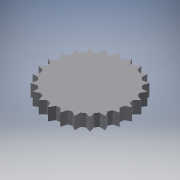
# Autodesk Inventor part: Piñon_1
Saved by Autodesk Inventor 2017 (Build 210142000, 142)
## iProperties
Part Number: Piñon_1
Material: Genérico
Document SubType Name: Modeling
Designer: Daniel Caycedo
Density: 1 g/cm^3
Appearance: Valor por defecto
Author: Daniel Caycedo
Autodesk Inventor part; units mm, degrees
ref_plane "YZ Plane" through (0, 0, 0) normal (1, 0, 0) x (0, 1, 0)
ref_plane "XZ Plane" through (0, 0, 0) normal (0, 1, 0) x (-1, 0, 0)
ref_plane "XY Plane" through (0, 0, 0) normal (0, 0, 1) x (1, 0, 0)
sketch "Boceto1" plane through (0, 0, 0) normal (0, 0, 1) x (1, 0, 0)
  circle A0 centre (0, 0) radius 15
  line L0 (0, 0) -> (0, 15)
  line L1 (0, 15) -> (0, 14)
  line L2 (-1.7321, 14) -> (0, 17)
  line L3 (0, 17) -> (1.7321, 14)
  line L4 (1.7321, 14) -> (-1.7321, 14)
  line L5 (-5.2965, 13.0747) -> (-4.3999, 16.4207)
  line L6 (-1.9504, 13.9712) -> (-5.2965, 13.0747)
  line L7 (-4.3999, 16.4207) -> (-1.9504, 13.9712)
  line L8 (-8.5, 11.2583) -> (-8.5, 14.7224)
  line L9 (-5.5, 12.9904) -> (-8.5, 11.2583)
  line L10 (-8.5, 14.7224) -> (-5.5, 12.9904)
  line L11 (-11.1242, 8.6748) -> (-12.0208, 12.0208)
  line L12 (-8.6748, 11.1242) -> (-11.1242, 8.6748)
  line L13 (-12.0208, 12.0208) -> (-8.6748, 11.1242)
  line L14 (-12.9904, 5.5) -> (-14.7224, 8.5)
  line L15 (-11.2583, 8.5) -> (-12.9904, 5.5)
  line L16 (-14.7224, 8.5) -> (-11.2583, 8.5)
  line L17 (-13.9712, 1.9504) -> (-16.4207, 4.3999)
  line L18 (-13.0747, 5.2965) -> (-13.9712, 1.9504)
  line L19 (-16.4207, 4.3999) -> (-13.0747, 5.2965)
  line L20 (-14, -1.7321) -> (-17, 0)
  line L21 (-14, 1.7321) -> (-14, -1.7321)
  line L22 (-17, 0) -> (-14, 1.7321)
  line L23 (-13.0747, -5.2965) -> (-16.4207, -4.3999)
  line L24 (-13.9712, -1.9504) -> (-13.0747, -5.2965)
  line L25 (-16.4207, -4.3999) -> (-13.9712, -1.9504)
  line L26 (-11.2583, -8.5) -> (-14.7224, -8.5)
  line L27 (-12.9904, -5.5) -> (-11.2583, -8.5)
  line L28 (-14.7224, -8.5) -> (-12.9904, -5.5)
  line L29 (-8.6748, -11.1242) -> (-12.0208, -12.0208)
  line L30 (-11.1242, -8.6748) -> (-8.6748, -11.1242)
  line L31 (-12.0208, -12.0208) -> (-11.1242, -8.6748)
  line L32 (-5.5, -12.9904) -> (-8.5, -14.7224)
  line L33 (-8.5, -11.2583) -> (-5.5, -12.9904)
  line L34 (-8.5, -14.7224) -> (-8.5, -11.2583)
  line L35 (-1.9504, -13.9712) -> (-4.3999, -16.4207)
  line L36 (-5.2965, -13.0747) -> (-1.9504, -13.9712)
  line L37 (-4.3999, -16.4207) -> (-5.2965, -13.0747)
  line L38 (1.7321, -14) -> (0, -17)
  line L39 (-1.7321, -14) -> (1.7321, -14)
  line L40 (0, -17) -> (-1.7321, -14)
  line L41 (5.2965, -13.0747) -> (4.3999, -16.4207)
  line L42 (1.9504, -13.9712) -> (5.2965, -13.0747)
  line L43 (4.3999, -16.4207) -> (1.9504, -13.9712)
  line L44 (8.5, -11.2583) -> (8.5, -14.7224)
  line L45 (5.5, -12.9904) -> (8.5, -11.2583)
  line L46 (8.5, -14.7224) -> (5.5, -12.9904)
  line L47 (11.1242, -8.6748) -> (12.0208, -12.0208)
  line L48 (8.6748, -11.1242) -> (11.1242, -8.6748)
  line L49 (12.0208, -12.0208) -> (8.6748, -11.1242)
  line L50 (12.9904, -5.5) -> (14.7224, -8.5)
  line L51 (11.2583, -8.5) -> (12.9904, -5.5)
  line L52 (14.7224, -8.5) -> (11.2583, -8.5)
  line L53 (13.9712, -1.9504) -> (16.4207, -4.3999)
  line L54 (13.0747, -5.2965) -> (13.9712, -1.9504)
  line L55 (16.4207, -4.3999) -> (13.0747, -5.2965)
  line L56 (14, 1.7321) -> (17, 0)
  line L57 (14, -1.7321) -> (14, 1.7321)
  line L58 (17, 0) -> (14, -1.7321)
  line L59 (13.0747, 5.2965) -> (16.4207, 4.3999)
  line L60 (13.9712, 1.9504) -> (13.0747, 5.2965)
  line L61 (16.4207, 4.3999) -> (13.9712, 1.9504)
  line L62 (11.2583, 8.5) -> (14.7224, 8.5)
  line L63 (12.9904, 5.5) -> (11.2583, 8.5)
  line L64 (14.7224, 8.5) -> (12.9904, 5.5)
  line L65 (8.6748, 11.1242) -> (12.0208, 12.0208)
  line L66 (11.1242, 8.6748) -> (8.6748, 11.1242)
  line L67 (12.0208, 12.0208) -> (11.1242, 8.6748)
  line L68 (5.5, 12.9904) -> (8.5, 14.7224)
  line L69 (8.5, 11.2583) -> (5.5, 12.9904)
  line L70 (8.5, 14.7224) -> (8.5, 11.2583)
  line L71 (1.9504, 13.9712) -> (4.3999, 16.4207)
  line L72 (5.2965, 13.0747) -> (1.9504, 13.9712)
  line L73 (4.3999, 16.4207) -> (5.2965, 13.0747)
  point P0 (-3.6235, 13.523)
  point P1 (-7, 12.1244)
  point P2 (-9.8995, 9.8995)
  point P3 (-12.1244, 7)
  point P4 (-13.523, 3.6235)
  point P5 (-14, 0)
  point P6 (-13.523, -3.6235)
  point P7 (-12.1244, -7)
  point P8 (-9.8995, -9.8995)
  point P9 (-7, -12.1244)
  point P10 (-3.6235, -13.523)
  point P11 (0, -14)
  point P12 (3.6235, -13.523)
  point P13 (7, -12.1244)
  point P14 (9.8995, -9.8995)
  point P15 (12.1244, -7)
  point P16 (13.523, -3.6235)
  point P17 (14, 0)
  point P18 (13.523, 3.6235)
  point P19 (12.1244, 7)
  point P20 (9.8995, 9.8995)
  point P21 (7, 12.1244)
  point P22 (3.6235, 13.523)
  dimension "d0" = 30
  dimension "d1" = 1
  dimension "d4" = 360
  constraints: 148 end point, 2 coincident, 1 midpoint, 1 point on line, 1 vertical, 1 vertical alignment, 178 other
  measures "d1" distance of L0.end L1.end
extrude "Extrusión1" add sketch "Boceto1" along normal blind 5
sketch "Boceto2" plane through (0, 0, 0) normal (0, 0, -1) x (-1, 0, 0)
  circle A0 centre (0, 0) radius 3
  line L0 (0, 0) -> (0, 3)
  line L1 (0, 3) -> (0, 2.8)
  line L2 (-0.3464, 2.8) -> (0, 3.4)
  line L3 (0, 3.4) -> (0.3464, 2.8)
  line L4 (0.3464, 2.8) -> (-0.3464, 2.8)
  line L5 (-0.88, 3.2841) -> (-0.3901, 2.7942)
  line L6 (-1.0593, 2.6149) -> (-0.88, 3.2841)
  line L7 (-0.3901, 2.7942) -> (-1.0593, 2.6149)
  line L8 (-1.7, 2.9445) -> (-1.1, 2.5981)
  line L9 (-1.7, 2.2517) -> (-1.7, 2.9445)
  line L10 (-1.1, 2.5981) -> (-1.7, 2.2517)
  line L11 (-2.4042, 2.4042) -> (-1.735, 2.2248)
  line L12 (-2.2248, 1.735) -> (-2.4042, 2.4042)
  line L13 (-1.735, 2.2248) -> (-2.2248, 1.735)
  line L14 (-2.9445, 1.7) -> (-2.2517, 1.7)
  line L15 (-2.5981, 1.1) -> (-2.9445, 1.7)
  line L16 (-2.2517, 1.7) -> (-2.5981, 1.1)
  line L17 (-3.2841, 0.88) -> (-2.6149, 1.0593)
  line L18 (-2.7942, 0.3901) -> (-3.2841, 0.88)
  line L19 (-2.6149, 1.0593) -> (-2.7942, 0.3901)
  line L20 (-3.4, 0) -> (-2.8, 0.3464)
  line L21 (-2.8, -0.3464) -> (-3.4, 0)
  line L22 (-2.8, 0.3464) -> (-2.8, -0.3464)
  line L23 (-3.2841, -0.88) -> (-2.7942, -0.3901)
  line L24 (-2.6149, -1.0593) -> (-3.2841, -0.88)
  line L25 (-2.7942, -0.3901) -> (-2.6149, -1.0593)
  line L26 (-2.9445, -1.7) -> (-2.5981, -1.1)
  line L27 (-2.2517, -1.7) -> (-2.9445, -1.7)
  line L28 (-2.5981, -1.1) -> (-2.2517, -1.7)
  line L29 (-2.4042, -2.4042) -> (-2.2248, -1.735)
  line L30 (-1.735, -2.2248) -> (-2.4042, -2.4042)
  line L31 (-2.2248, -1.735) -> (-1.735, -2.2248)
  line L32 (-1.7, -2.9445) -> (-1.7, -2.2517)
  line L33 (-1.1, -2.5981) -> (-1.7, -2.9445)
  line L34 (-1.7, -2.2517) -> (-1.1, -2.5981)
  line L35 (-0.88, -3.2841) -> (-1.0593, -2.6149)
  line L36 (-0.3901, -2.7942) -> (-0.88, -3.2841)
  line L37 (-1.0593, -2.6149) -> (-0.3901, -2.7942)
  line L38 (0, -3.4) -> (-0.3464, -2.8)
  line L39 (0.3464, -2.8) -> (0, -3.4)
  line L40 (-0.3464, -2.8) -> (0.3464, -2.8)
  line L41 (0.88, -3.2841) -> (0.3901, -2.7942)
  line L42 (1.0593, -2.6149) -> (0.88, -3.2841)
  line L43 (0.3901, -2.7942) -> (1.0593, -2.6149)
  line L44 (1.7, -2.9445) -> (1.1, -2.5981)
  line L45 (1.7, -2.2517) -> (1.7, -2.9445)
  line L46 (1.1, -2.5981) -> (1.7, -2.2517)
  line L47 (2.4042, -2.4042) -> (1.735, -2.2248)
  line L48 (2.2248, -1.735) -> (2.4042, -2.4042)
  line L49 (1.735, -2.2248) -> (2.2248, -1.735)
  line L50 (2.9445, -1.7) -> (2.2517, -1.7)
  line L51 (2.5981, -1.1) -> (2.9445, -1.7)
  line L52 (2.2517, -1.7) -> (2.5981, -1.1)
  line L53 (3.2841, -0.88) -> (2.6149, -1.0593)
  line L54 (2.7942, -0.3901) -> (3.2841, -0.88)
  line L55 (2.6149, -1.0593) -> (2.7942, -0.3901)
  line L56 (3.4, 0) -> (2.8, -0.3464)
  line L57 (2.8, 0.3464) -> (3.4, 0)
  line L58 (2.8, -0.3464) -> (2.8, 0.3464)
  line L59 (3.2841, 0.88) -> (2.7942, 0.3901)
  line L60 (2.6149, 1.0593) -> (3.2841, 0.88)
  line L61 (2.7942, 0.3901) -> (2.6149, 1.0593)
  line L62 (2.9445, 1.7) -> (2.5981, 1.1)
  line L63 (2.2517, 1.7) -> (2.9445, 1.7)
  line L64 (2.5981, 1.1) -> (2.2517, 1.7)
  line L65 (2.4042, 2.4042) -> (2.2248, 1.735)
  line L66 (1.735, 2.2248) -> (2.4042, 2.4042)
  line L67 (2.2248, 1.735) -> (1.735, 2.2248)
  line L68 (1.7, 2.9445) -> (1.7, 2.2517)
  line L69 (1.1, 2.5981) -> (1.7, 2.9445)
  line L70 (1.7, 2.2517) -> (1.1, 2.5981)
  line L71 (0.88, 3.2841) -> (1.0593, 2.6149)
  line L72 (0.3901, 2.7942) -> (0.88, 3.2841)
  line L73 (1.0593, 2.6149) -> (0.3901, 2.7942)
  point P0 (-0.7247, 2.7046)
  point P1 (-1.4, 2.4249)
  point P2 (-1.9799, 1.9799)
  point P3 (-2.4249, 1.4)
  point P4 (-2.7046, 0.7247)
  point P5 (-2.8, 0)
  point P6 (-2.7046, -0.7247)
  point P7 (-2.4249, -1.4)
  point P8 (-1.9799, -1.9799)
  point P9 (-1.4, -2.4249)
  point P10 (-0.7247, -2.7046)
  point P11 (0, -2.8)
  point P12 (0.7247, -2.7046)
  point P13 (1.4, -2.4249)
  point P14 (1.9799, -1.9799)
  point P15 (2.4249, -1.4)
  point P16 (2.7046, -0.7247)
  point P17 (2.8, 0)
  point P18 (2.7046, 0.7247)
  point P19 (2.4249, 1.4)
  point P20 (1.9799, 1.9799)
  point P21 (1.4, 2.4249)
  point P22 (0.7247, 2.7046)
  dimension "d8" = 6
  dimension "d9" = 0.2
  dimension "d12" = 360
  constraints: 148 end point, 2 coincident, 1 midpoint, 1 point on line, 1 vertical, 1 vertical alignment, 178 other
  measures "d9" distance of L0.end L1.end
extrude "Extrusión2" cut sketch "Boceto2" against normal blind 5
